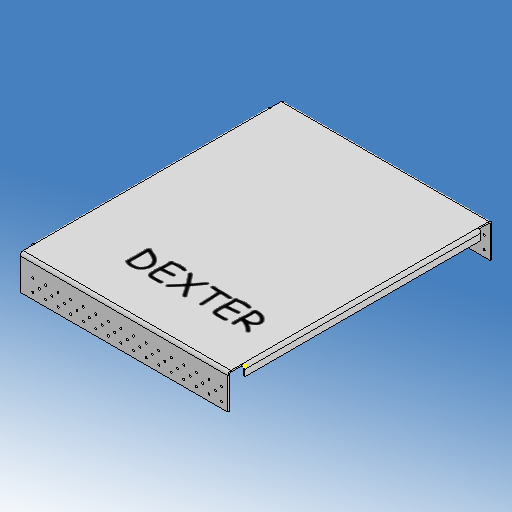
# Autodesk Inventor part: EBoxCover
Saved by Autodesk Inventor 2025 (Build 290162000, 162)
## iProperties
Created: 2024-06-27
Part Number: EBoxCover
Material: Generic
Document SubType Name: Sheet Metal
Designer: seene
Density: 1 g/cm^3
Sheet Metal Rule: Default
Appearance: Default
Author: seene
Autodesk Inventor part; units mm, degrees
ref_plane "YZ Plane" through (0, 0, 0) normal (1, 0, 0) x (0, 1, 0)
ref_plane "XZ Plane" through (0, 0, 0) normal (0, 1, 0) x (-1, 0, 0)
ref_plane "XY Plane" through (0, 0, 0) normal (0, 0, 1) x (1, 0, 0)
sketch "Sketch1" plane through (0, 0, 0) normal (0, 1, 0) x (-1, 0, 0)
  line L0 (0, 0) -> (431.8, 0)
  line L1 (431.8, 0) -> (431.8, -476.504)
  line L2 (431.8, -476.504) -> (0, -476.504)
  line L3 (0, -476.504) -> (0, 0)
  dimension "d0" = 431.8
  dimension "d1" = 476.504
  measures "d0" distance of L1.end L2.end
  measures "d1" distance between parallel lines of L2 L0
extrude "Plate1" add sketch "Sketch1" along normal blind 3.048
sketch "Sketch3" plane through (-3.048, 3.048, 0) normal (1, 0, 0) x (0, 1, 0)
  line L0 (0, -476.504) -> (0, 0)
  line L1 (0, 0) -> (-19.05, 0)
  line L2 (-19.05, 0) -> (-19.05, -476.504)
  line L3 (-19.05, -476.504) -> (0, -476.504)
  constraints: 6 end point, 1 horizontal, 1 perpendicular, 1 vertical
edge flange "Flange2" height 19.05 angle 90 thickness 3.048 bend radius 3.048 thickness toward (1, 0, 0) relief straight relief width 3.048 relief depth 1.524 corner gap 3.048 corner form 0 edges at (0, 0, -238.252) (-431.8, 0, -238.252) wall of the first edge with corners at (-3.048, 3.048, -476.504) (-3.048, 3.048, 0) (-3.048, -16.002, 0) (-3.048, -16.002, -476.504)
bend "Bend2"
corner "Corner2"
sketch "Sketch5" plane through (0, 0, 0) normal (0, -1, 0) x (1, 0, 0)
  line L0 (-425.704, 0) -> (-425.704, -476.504)
  line L1 (-6.096, -476.504) -> (-6.096, 0)
  line L2 (-6.096, -476.504) -> (-425.704, -476.504)
  line L3 (-425.704, 0) -> (-6.096, 0)
  line L4 (-425.704, 28.448) -> (-6.096, 28.448)
  line L5 (-6.096, 28.448) -> (-6.096, -504.952)
  line L6 (-6.096, -504.952) -> (-425.704, -504.952)
  line L7 (-425.704, -504.952) -> (-425.704, 28.448)
  line L8 (-425.704, -238.252) -> (-6.096, -238.252) construction
  line L9 (-425.704, -238.252) -> (-6.096, -238.252) construction
  line L10 (-425.704, -476.504) -> (-425.704, 0) construction
  line L11 (-6.096, 0) -> (-6.096, -476.504) construction
  point P0 (-6.096, -476.504)
  point P1 (-425.704, -476.504)
  point P2 (-425.704, 0)
  dimension "d63" = 533.4
  measures "d63" distance of L4.end L5.end
sheet face with bend "Face2" sketch "Sketch5" thickness 3.048 toward (0, 1, 0) bend radius 3.048 relief straight relief width 3.048 relief depth 1.524 contours L7 L4 L5 L3 | L2 L5 L6 L7
bend "Bend3"
sketch "Sketch6" plane through (-425.704, 3.048, 25.4) normal (0, 0, 1) x (1, 0, 0)
  line L0 (419.608, 0) -> (0, 0)
  line L1 (0, 0) -> (0, -69.85)
  line L2 (0, -69.85) -> (419.608, -69.85)
  line L3 (419.608, -69.85) -> (419.608, 0)
  constraints: 6 end point, 1 horizontal, 1 perpendicular, 1 vertical
edge flange "Flange3" height 69.85 angle 90 thickness 3.048 bend radius 3.048 thickness toward (0, 0, 1) relief straight relief width 3.048 relief depth 1.524 corner gap 3.048 corner form 0 edges at (-215.9, 0, 28.448) (-215.9, 0, -504.952) wall of the first edge with corners at (-6.096, 3.048, 25.4) (-425.704, 3.048, 25.4) (-425.704, -66.802, 25.4) (-6.096, -66.802, 25.4)
bend "Bend4"
corner "Corner3"
sketch "Sketch4" plane through (-431.8, -66.802, 28.448) normal (0, 0, 1) x (1, 0, 0)
  circle A0 centre (413.004, 38.1) radius 2.0701
  circle A1 centre (413.004, 12.7) radius 2.0701
  circle A2 centre (387.604, 12.7) radius 2.0701
  circle A3 centre (387.604, 38.1) radius 2.0701
  circle A4 centre (400.304, 25.4) radius 2.0701
  line L0 (387.604, 38.1) -> (413.004, 12.7) construction
  line L1 (413.004, 12.7) -> (387.604, 12.7) construction
  line L2 (387.604, 12.7) -> (413.004, 38.1) construction
  line L3 (381, 0) -> (0, 0) construction
  line L4 (425.704, 63.754) -> (425.704, 0) projected
  point P0 (381, 66.802)
  dimension "d23" = 4.1402
  dimension "d25" = 25.4
  dimension "d26" = 25.4
  dimension "d28" = 12.7
  dimension "d64" = 12.7
  constraints: 6 end point, 5 centre point, 4 equal radius, 2 horizontal alignment, 2 vertical alignment, 1 horizontal, 1 midpoint
  measures "d23" diameter of A4
  measures "d25" distance of L2.end L0.start
  measures "d26" distance of L1.end L0.start
  measures "d28" distance from line of L3 L0.end
  measures "d64" distance from line of L4 L2.end
extrude "Extrusion2" cut sketch "Sketch4" against normal through all
pattern_linear "Rectangular Pattern4" count 15 spacing 25.4 along (-1, 0, 0) of "Extrusion2"
sketch "Sketch7" plane through (0, 3.048, 0) normal (0, 1, 0) x (1, 0, 0)
  line L0 (-309.923, 111.4622) -> (-59.4634, 111.4622) construction
  line L1 (-59.4634, 111.4622) -> (-59.4634, 177.8246) construction
  line L2 (-59.4634, 177.8246) -> (-309.923, 177.8246) construction
  line L3 (-309.923, 177.8246) -> (-309.923, 111.4622) construction
  point P0 (0, 0)
  constraints: 2 other
equation "\"d2\" = Thickness"
equation "\"d13\" = BendReliefWidth"
equation "\"d14\" = BendReliefDepth"
equation "\"d15\" = MinimumRemnant"
equation "\"d16\" = TransitionRadius"
equation "\"d19\" = BendRadius"
equation "\"d20\" = CornerReliefSize"
equation "\"d21\" = GapSize"
equation "\"d22\" = JacobiRadiusSize"
equation "\"d36\" = BendRadius"
equation "\"d37\" = BendReliefWidth"
equation "\"d39\" = MinimumRemnant"
equation "\"d38\" = BendReliefDepth"
equation "\"d40\" = TransitionRadius"
equation "\"d41\" = BendReliefWidth"
equation "\"d42\" = BendReliefDepth"
equation "\"d43\" = MinimumRemnant"
equation "\"d44\" = TransitionRadius"
equation "\"d47\" = BendRadius"
equation "\"d48\" = CornerReliefSize"
equation "\"d49\" = GapSize"
equation "\"d50\" = JacobiRadiusSize"
equation "\"BendRadius\" = Thickness"
equation "\"BendReliefWidth\" = Thickness"
equation "\"BendReliefDepth\" = 0.5 * Thickness"
equation "\"CornerReliefSize\" = 4 * Thickness"
equation "\"MinimumRemnant\" = 2 * Thickness"
equation "\"TransitionRadius\" = BendRadius"
equation "\"JacobiRadiusSize\" = BendRadius"
equation "\"GapSize\" = Thickness"
equation "\"Thickness\" = 3.048"
body "Solid1"
